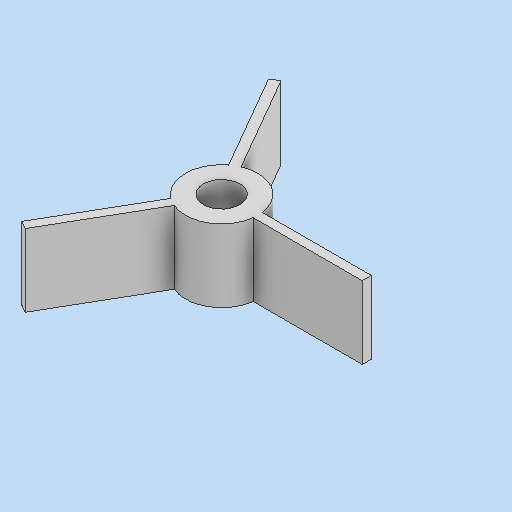
# Autodesk Inventor part: brush_tpu_test_print
Saved by Autodesk Inventor 2026 (Build 300175000, 175)
## iProperties
Created: 2026-02-09
Part Number: brush_tpu_test_print
Material: Generic
Document SubType Name: Modeling
Designer: mones
Density: 1 g/cm^3
Appearance: Default
Author: mones
Autodesk Inventor part; units mm, degrees
ref_plane "YZ Plane" through (0, 0, 0) normal (1, 0, 0) x (0, 1, 0)
ref_plane "XZ Plane" through (0, 0, 0) normal (0, 1, 0) x (-1, 0, 0)
ref_plane "XY Plane" through (0, 0, 0) normal (0, 0, 1) x (1, 0, 0)
sketch "Sketch1" plane through (0, 0, 0) normal (0, 1, 0) x (-1, 0, 0)
  circle A0 centre (0, 0) radius 6.35
  circle A1 centre (0, 0) radius 3.175
  line L0 (0, 0) -> (-25.4, 0)
  line L1 (0, 0) -> (12.7, -21.997)
  line L2 (0, 0) -> (12.7, 21.997)
  line L3 (12.0126, 22.3939) -> (13.3874, 21.6002)
  line L4 (13.3874, 21.6002) -> (-0.6874, 0.3969) construction
  line L5 (0.6874, -0.3969) -> (12.0126, 22.3939) construction
  line L6 (-25.4, 0.7937) -> (-25.4, -0.7937)
  line L7 (0, -0.7937) -> (0, 0)
  line L8 (0, 0.7937) -> (-25.4, -0.7937) construction
  line L9 (-25.4, 0.7937) -> (0, -0.7937) construction
  line L10 (13.3874, -21.6002) -> (12.0126, -22.3939)
  line L11 (0.6874, 0.3969) -> (12.0126, -22.3939) construction
  line L12 (13.3874, -21.6002) -> (-0.6874, -0.3969) construction
  line L13 (-25.4, -0.7937) -> (-3.0742, -0.7937)
  line L14 (-3.0742, 0.7937) -> (-25.4, 0.7937)
  line L15 (0.8497, 3.0592) -> (12.0126, 22.3939)
  line L16 (13.3874, 21.6002) -> (2.2245, 2.2654)
  line L17 (2.2245, -2.2654) -> (13.3874, -21.6002)
  line L18 (12.0126, -22.3939) -> (0.8497, -3.0592)
  point P0 (6.35, 10.9985)
  point P1 (-12.7, 0)
  point P2 (6.35, -10.9985)
  point P3 (3.8375, -5.0593)
  point P4 (3.175, -5.4993)
  point P5 (-6.3002, -0.7937)
  point P6 (2.4627, -5.853)
  point P7 (3.8375, 5.0593)
  point P8 (2.4627, 5.853)
  point P9 (-6.3002, 0.7938)
  dimension "d5" = 360
  constraints: 38 end point, 9 midpoint, 6 parallel, 6 point on circle, 2 centre point, 2 perpendicular, 1 coincident, 1 horizontal, 7 other
extrude "Extrusion1" add sketch "Sketch1" along normal blind 12.7 contours A0 L17 A1 L16 | L16 A1 L2 A0 | A0 L2 L3 L16 | L17 L10 L1 A0 | A0 L1 A1 L17 | L2 A1 L15 A0 | A0 L15 L3 L2 | L1 L10 L18 A0 | A0 L18 A1 L1 | L15 A1 L14 A0 | A0 L13 A1 L18 | L14 A1 L0 A0 | A0 L0 L6 L14 | L13 L6 L0 A0 | A0 L0 A1 L13
body "Solid1"
